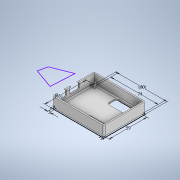
# Autodesk Inventor part: Boks_V2
Saved by Autodesk Inventor 2022 (Build 260153000, 153)
## iProperties
Created: 2021-08-17
Part Number: Boks_V2
Material: Generic
Document SubType Name: Modeling
Designer: Bruker
Density: 1 g/cm^3
Appearance: Default
Author: Bruker
Autodesk Inventor part; units mm, degrees
ref_plane "YZ Plane" through (0, 0, 0) normal (1, 0, 0) x (0, 1, 0)
ref_plane "XZ Plane" through (0, 0, 0) normal (0, 1, 0) x (-1, 0, 0)
ref_plane "XY Plane" through (0, 0, 0) normal (0, 0, 1) x (1, 0, 0)
sketch "Sketch1" plane through (0, 0, 0) normal (0, 1, 0) x (-1, 0, 0)
  line L0 (0, 0) -> (74, 0)
  line L1 (74, 0) -> (74, -59)
  line L2 (74, -59) -> (0, -59)
  line L3 (0, -59) -> (0, 0)
  line L4 (77, 3) -> (-3, 3)
  line L5 (-3, 3) -> (-3, -62)
  line L6 (-3, -62) -> (77, -62)
  line L7 (77, -62) -> (77, 3)
  line L8 (107, -62) -> (109, -25)
  line L9 (109, -25) -> (140, -36)
  line L10 (140, -36) -> (137, -50)
  line L11 (137, -50) -> (107, -62)
  dimension "d0" = 74
  dimension "d1" = 59
  dimension "d2" = 3
  dimension "d3" = 3
  dimension "d4" = 65
  dimension "d5" = 3
  dimension "d6" = 3
  dimension "d7" = 80
  constraints: 24 end point, 4 parallel, 2 horizontal, 2 perpendicular
  measures "d0" distance of L1.end L2.end
  measures "d1" distance of L2.end L0.start
  measures "d2" distance between parallel lines of L6 L2
  measures "d3" distance between parallel lines of L0 L4
  measures "d4" distance of L6.end L4.start
  measures "d5" distance between parallel lines of L1 L7
  measures "d6" distance between parallel lines of L3 L5
  measures "d7" distance of L5.end L6.end
extrude "Grunnflate" add sketch "Sketch1" along normal blind 2 contours L0 L1 L2 L3 | L7 L6 L5 L4
sketch "Sketch2" plane through (0, 2, 0) normal (0, 1, 0) x (1, 0, 0)
  circle A0 centre (-71.5, 2.5) radius 2.5
  circle A1 centre (-71.5, 56.5) radius 2.5
  circle A2 centre (-2.5, 2.5) radius 3
  circle A3 centre (-2.5, 56.5) radius 3
  line L0 (0, 59) -> (-74, 59)
  line L1 (-74, 59) -> (-74, 0)
  line L2 (-74, 0) -> (0, 0)
  line L3 (0, 0) -> (0, 59)
  line L4 (-77, 62) -> (-77, -3) projected
  line L5 (3, 62) -> (-77, 62) projected
  line L6 (3, -3) -> (3, 62) projected
  line L7 (-77, -3) -> (3, -3) projected
  point P0 (0, 0)
  dimension "d10" = 6
  dimension "d11" = 6
  dimension "d12" = 5
  dimension "d13" = 5
  dimension "d14" = 3
  dimension "d15" = 3
  dimension "d16" = 3
  dimension "d17" = 3
  dimension "d19" = 2.5
  dimension "d20" = 2.5
  dimension "d21" = 2.5
  dimension "d22" = 2.5
  dimension "d23" = 2.5
  dimension "d24" = 2.5
  dimension "d26" = 2.5
  dimension "d27" = 54
  dimension "d76" = 2.5
  constraints: 8 end point, 4 centre point, 2 parallel, 1 horizontal, 1 perpendicular
  measures "d10" diameter of A2
  measures "d11" diameter of A3
  measures "d12" diameter of A0
  measures "d13" diameter of A1
  measures "d14" distance between parallel lines of L4 L1
  measures "d15" distance between parallel lines of L5 L0
  measures "d16" distance between parallel lines of L6 L3
  measures "d17" distance between parallel lines of L7 L2
  measures "d19" distance from line of L1 A1.centre
  measures "d20" distance from line of L0 A1.centre
  measures "d21" distance from line of L0 A3.centre
  measures "d22" distance from line of L3 A2.centre
  measures "d23" distance from line of L2 A2.centre
  measures "d24" distance from line of L1 A0.centre
  measures "d26" distance from line of L2 A0.centre
  measures "d27" distance of A0.centre A1.centre
  measures "d76" distance from line of L3 A3.centre
extrude "Suport" add sketch "Sketch2" along normal blind 6 contours A0 | A1 | L2 A2 | A2 L3 L2 | A2 L3 | L0 A3 L3 | A3 L0 | L3 A3 picked at (-1.9986, 1.7181) picked at (-2.4592, 57.1675)
sketch "Sketch3" plane through (-71.5, 8, -2.5) normal (0, 1, 0) x (1, 0, 0)
  circle A0 centre (0, 0) radius 1
  circle A1 centre (0, 54) radius 2.5 projected
  circle A2 centre (0, 54) radius 1
  circle A3 centre (69, 54) radius 3 projected
  circle A4 centre (69, 54) radius 1.5
  circle A5 centre (69, 0) radius 3 projected
  circle A6 centre (69, 0) radius 1.5
  point P0 (71.5, -2.5)
  dimension "d30" = 2
  dimension "d31" = 2
  dimension "d32" = 3
  dimension "d33" = 3
  constraints: 4 centre point, 3 coincident
  measures "d30" diameter of A0
  measures "d31" diameter of A2
  measures "d32" diameter of A6
  measures "d33" diameter of A4
extrude "Skruehull" cut sketch "Sketch3" against normal blind 32 contours A0 | A2 | A4 | A6
sketch "Sketch4" plane through (0, 2, 0) normal (0, 1, 0) x (1, 0, 0)
  line L0 (-9, 0) -> (-39, 0)
  line L1 (-39, 0) -> (-39, 15)
  line L2 (-39, 15) -> (-9, 15)
  line L3 (-9, 15) -> (-9, 0)
  line L4 (-9, 44) -> (-39, 44)
  line L5 (-39, 44) -> (-39, 59)
  line L6 (-39, 59) -> (-9, 59)
  line L7 (-9, 59) -> (-9, 44)
  line L8 (-77, -3) -> (3, -3) projected
  line L9 (3, 62) -> (-77, 62) projected
  line L10 (3, -3) -> (3, 62) projected
  point P0 (0, 0)
  dimension "d36" = 15
  dimension "d37" = 15
  dimension "d38" = 3
  dimension "d39" = 3
  dimension "d40" = 30
  dimension "d41" = 12
  constraints: 16 end point, 4 parallel, 2 horizontal, 2 perpendicular, 2 point on line
  measures "d36" distance of L0.end L1.end
  measures "d37" distance of L4.end L5.end
  measures "d38" distance between parallel lines of L8 L0
  measures "d39" distance between parallel lines of L9 L6
  measures "d40" distance of L5.end L6.end
  measures "d41" distance between parallel lines of L10 L7
extrude "Bunnhull" cut sketch "Sketch4" against normal blind 38
sketch "Sketch5" plane through (0, 2, 0) normal (0, 1, 0) x (1, 0, 0)
  line L0 (1, -1) -> (-75, -1)
  line L1 (-75, -1) -> (-75, 60)
  line L2 (-75, 60) -> (1, 60)
  line L3 (1, 60) -> (1, -1)
  line L4 (-77, 62) -> (-77, -3) projected
  line L5 (3, 62) -> (-77, 62) projected
  line L6 (3, -3) -> (3, 62) projected
  line L7 (-77, -3) -> (3, -3) projected
  point P0 (0, 0)
  dimension "d44" = 2
  dimension "d45" = 2
  dimension "d46" = 2
  dimension "d47" = 2
  constraints: 8 end point, 2 parallel, 1 horizontal, 1 perpendicular
  measures "d44" distance between parallel lines of L4 L1
  measures "d45" distance between parallel lines of L5 L2
  measures "d46" distance between parallel lines of L6 L3
  measures "d47" distance between parallel lines of L7 L0
extrude "Vegger" add sketch "Sketch5" along normal blind 15
sketch "Sketch6" plane through (-77, 0, -62) normal (-1, 0, 0) x (0, 0, 1)
  line L0 (45, 7) -> (60, 7)
  line L1 (60, 7) -> (60, 17)
  line L2 (60, 17) -> (45, 17)
  line L3 (45, 17) -> (45, 7)
  line L4 (65, 0) -> (65, 17) projected
  line L5 (0, 17) -> (65, 17) projected
  line L6 (0, 0) -> (65, 0) projected
  point P0 (62, 0)
  dimension "d50" = 15
  dimension "d51" = 10
  dimension "d52" = 5
  dimension "d53" = 0
  dimension "d54" = 7
  constraints: 8 end point, 2 parallel, 1 horizontal, 1 perpendicular
  measures "d50" distance of L1.end L2.end
  measures "d51" distance of L0.end L1.end
  measures "d52" distance between parallel lines of L4 L1
  measures "d53" distance between parallel lines of L5 L2
  measures "d54" distance between parallel lines of L6 L0
extrude "USB-inn" cut sketch "Sketch6" against normal blind 2
fillet "Fillet1" radius 2 8 edges at (-77, 8.5, 3) (-77, 8.5, -62) (3, 8.5, -62) (3, 8.5, 3) (3, 0, -29.5) (-37, 0, 3) (-77, 0, -29.5) (-37, 0, -62)
fillet "Fillet2" radius 2 4 edges at (-37, 2, -60) (-75, 2, -29.5) (-37, 2, 1) (1, 2, -29.5)
fillet "Fillet3" radius 4 8 edges at (-39, 1, -44) (-39, 1.134, 0) (-39, 1, -15) (-39, 1.134, -59) (-9, 1, -44) (-9, 1.134, 0) (-9, 1.134, -59) (-9, 1, -15)
fillet "Fillet4" radius 2 2 edges at (-76, 7, -17) (-76, 7, -2)
sketch "Sketch7" plane through (0, 17, 0) normal (0, 1, 0) x (1, 0, 0)
  line L0 (-74.8167, 18.7697) -> (-78.1163, 18.7697)
  line L1 (-78.1163, 18.7697) -> (-78.1163, 0.3143)
  line L2 (-78.1163, 0.3143) -> (-74.8167, 0.3143)
  line L3 (-74.8167, 0.3143) -> (-74.8167, 18.7697)
  point P0 (0, 0)
  constraints: 8 end point, 2 parallel, 1 horizontal, 1 perpendicular
extrude "+Temp" add sketch "Sketch7" along normal blind 2
fillet "Fillet5" radius 2 2 edges at (-76, 17, -2) (-76, 17, -17)
sketch "Sketch8" plane through (0, 19, 0) normal (0, 1, 0) x (1, 0, 0)
  line L0 (-77, 18.7697) -> (-78.1163, 18.7697) projected
  line L1 (-75, 0.3143) -> (-74.8167, 0.3143) projected
  line L2 (-78.1163, 18.7697) -> (-74.8167, 18.7697)
  line L3 (-74.8167, 18.7697) -> (-74.8167, 0.3143)
  line L4 (-74.8167, 0.3143) -> (-78.1163, 0.3143)
  line L5 (-78.1163, 0.3143) -> (-78.1163, 18.7697)
  point P0 (0, 0)
  constraints: 8 end point, 2 parallel, 1 horizontal, 1 perpendicular
extrude "-Temp" cut sketch "Sketch8" against normal blind 2
sketch "Sketch9" plane through (-77, 2, 1) normal (-1, 0, 0) x (0, 0, 1)
  line L0 (-61, 15) -> (0, 15) projected
  line L1 (-38, 15) -> (-23, 15)
  line L2 (-23, 15) -> (-23, 5)
  line L3 (-23, 5) -> (-38, 5)
  line L4 (-38, 5) -> (-38, 15)
  line L5 (-63, 15) -> (-63, 0) projected
  line L6 (2, 0) -> (2, 15) projected
  line L7 (-5, 5) -> (-16, 5) projected
  point P0 (-1, -2)
  dimension "d66" = 40
  dimension "d67" = 40
  dimension "d68" = 0
  constraints: 8 end point, 2 parallel, 1 horizontal, 1 perpendicular, 1 point on line
  measures "d66" distance between parallel lines of L5 L2
  measures "d67" distance between parallel lines of L6 L4
  measures "d68" distance between parallel lines of L7 L3
extrude "LED-view" cut sketch "Sketch9" against normal blind 2
sketch "Sketch10" plane through (0, 17, 0) normal (0, 1, 0) x (1, 0, 0)
  line L0 (-73, 4.5) -> (-73, 54.5) projected
  line L1 (-73, 40.4014) -> (-82.0701, 40.4014)
  line L2 (-82.0701, 40.4014) -> (-82.0701, 18.2719)
  line L3 (-82.0701, 18.2719) -> (-73, 18.2719)
  line L4 (-73, 18.2719) -> (-73, 40.4014)
  point P0 (0, 0)
  constraints: 8 end point, 2 parallel, 1 horizontal, 1 perpendicular, 1 point on line
extrude "+Temp2" add sketch "Sketch10" along normal blind 2
fillet "Fillet6" radius 2 4 edges at (-76, 17, -37) (-76, 17, -22) (-76, 7, -37) (-76, 7, -22)
sketch "Sketch11" plane through (0, 19, 0) normal (0, 1, 0) x (1, 0, 0)
  line L0 (-70.5437, 43.4678) -> (-90.0148, 43.4678)
  line L1 (-90.0148, 43.4678) -> (-90.0148, 13.5464)
  line L2 (-90.0148, 13.5464) -> (-70.5437, 13.5464)
  line L3 (-70.5437, 13.5464) -> (-70.5437, 43.4678)
  point P0 (0, 0)
  constraints: 8 end point, 2 parallel, 1 horizontal, 1 perpendicular
extrude "Extrusion11" cut sketch "Sketch11" against normal blind 2
body "Solid1"
